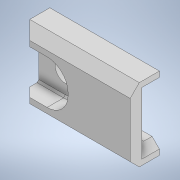
# Autodesk Inventor part: BatteryHolderFixture
Saved by Autodesk Inventor 2022 (Build 260153000, 153)
## iProperties
Created: 2021-04-26
Part Number: BatteryHolderFixture
Material: Generic
Document SubType Name: Modeling
Designer: lgnds
Density: 1 g/cm^3
Appearance: Default
Author: lgnds
## iProperties of the stored document BatteryHolderFixture_3DPrint.ipt
Created: 2021-04-26
Part Number: BatteryHolderFixture_3DPrint
Material: Generic
Document SubType Name: Modeling
Designer: lgnds
Density: 1 g/cm^3
Appearance: Default
Author: lgnds
Autodesk Inventor part; units mm, degrees
ref_plane "YZ Plane" through (0, 0, 0) normal (1, 0, 0) x (0, 1, 0)
ref_plane "XZ Plane" through (0, 0, 0) normal (0, 1, 0) x (-1, 0, 0)
ref_plane "XY Plane" through (0, 0, 0) normal (0, 0, 1) x (1, 0, 0)
sketch "Sketch1" plane through (0, 0, 0) normal (0, 0, 1) x (1, 0, 0)
  line L0 (-15, -10) -> (15, -10)
  line L1 (15, -10) -> (15, 10)
  line L2 (15, 10) -> (-15, 10)
  line L3 (-15, 10) -> (-15, -10)
  line L4 (-15, -10) -> (15, 10) construction
  line L5 (15, -10) -> (-15, 10) construction
  point P0 (0, 0)
  dimension "d0" = 20
  dimension "d1" = 30
  constraints: 12 end point, 2 midpoint, 2 parallel, 1 horizontal, 1 perpendicular
  measures "d0" distance between parallel lines of L0 L2
  measures "d1" distance between parallel lines of L3 L1
extrude "Extrusion1" add sketch "Sketch1" along normal blind 8
sketch "Sketch2" plane through (15, -10, 0) normal (1, 0, 0) x (0, 0, -1)
  line L0 (-9.6, 10) -> (1.6, 10) projected
  line L1 (0, 0) -> (0, 20) projected
  line L2 (0, 3.5) -> (-2.8, 3.5)
  line L3 (-2.8, 3.5) -> (-2.8, 16.5)
  line L4 (-2.8, 16.5) -> (0, 16.5)
  line L5 (0, 16.5) -> (0, 3.5)
  point P0 (0, 10)
  point P1 (0, 16.5)
  dimension "d4" = 2.8
  dimension "d5" = 13
  dimension "d6" = 6.5
  constraints: 8 end point, 2 parallel, 1 horizontal, 1 perpendicular, 1 point on line
  measures "d4" distance between parallel lines of L3 L1
  measures "d5" distance between parallel lines of L4 L2
  measures "d6" distance between parallel lines of L0 L2
extrude "Extrusion2" cut sketch "Sketch2" against normal blind 15
chamfer "Chamfer1" distance 2 angle 45 3 edges at (15, 0, 2.8) (15, 6.5, 1.4) (15, -6.5, 1.4)
chamfer "Chamfer2" distance 0.5 angle 45 2 edges at (6.5, 6.5, 2.8) (6.5, -6.5, 2.8)
sketch "Sketch3" plane through (0, 0, 8) normal (0, 0, 1) x (1, 0, 0)
  line L0 (-21, 0) -> (21, 0) projected
  line L1 (-2, -6) -> (-15, -6)
  line L2 (-15, -6) -> (-15, 6)
  line L3 (-15, 6) -> (-2, 6)
  line L4 (-2, 6) -> (-2, -6)
  line L5 (-2, -6) -> (-15, 6) construction
  line L6 (-15, -6) -> (-2, 6) construction
  line L7 (-15, 10) -> (-15, -10) projected
  line L8 (0, -6) -> (0, 6) projected
  point P0 (0, 0)
  point P1 (-8.5, 0)
  dimension "d15" = 2
  dimension "d16" = 12
  constraints: 12 end point, 2 midpoint, 2 parallel, 2 point on line, 1 horizontal, 1 perpendicular
  measures "d15" distance between parallel lines of L8 L4
  measures "d16" distance between parallel lines of L1 L3
extrude "Extrusion3" cut sketch "Sketch3" against normal blind 5
chamfer "Chamfer3" distance 2.5 angle 45 2 edges at (0, 10, 8) (0, -10, 8)
fillet "Fillet1" radius 5.75 2 edges at (-2, 6, 5.5) (-2, -6, 5.5)
chamfer "Chamfer4" distance 2.5 angle 45 2 edges at (-15, -6.75, 8) (-15, 6.75, 8)
sketch "Sketch4" plane through (0, 0, 3) normal (0, 0, 1) x (1, 0, 0)
  line L0 (-21, 0) -> (21, 0) projected
  circle A0 centre (-7.75, 0) radius 2.8
  arc A1 (-2, 0.25) -> (-7.75, 6) centre (-7.75, 0.25) ccw projected
  line L1 (-7.75, -6) -> (-15, -6) projected
  line L2 (-7.75, 6) -> (-7.75, -6) construction
  point P0 (0, 0)
  dimension "d26" = 5.6
  dimension "d27" = 0
  constraints: 2 end point, 1 centre point, 1 point on line, 1 vertical
  measures "d26" diameter of A0
  measures "d27" distance from line of A0.centre L2
extrude "Extrusion4" cut sketch "Sketch4" against normal blind 5
chamfer "Chamfer5" distance 0.5 angle 45 5 edges at (-3.6841, 4.3159, 3) (-11.375, 6, 3) (-2, 0, 3) (-3.6841, -4.3159, 3) (-11.375, -6, 3)
equation "\"d6\" = 0.5 * d5"
body "Solid1"
